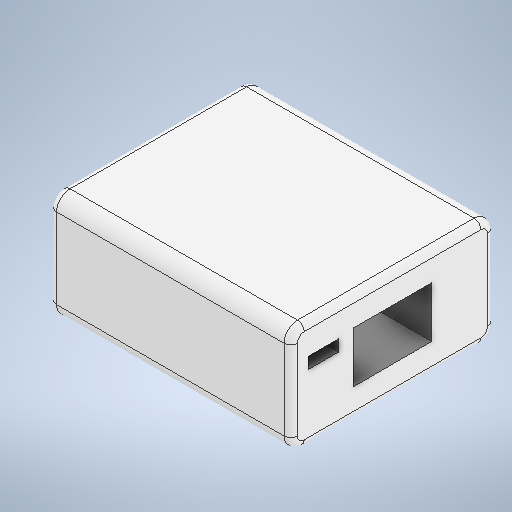
# Autodesk Inventor part: PoEbox
Saved by Autodesk Inventor 2025 (Build 290162000, 162)
## iProperties
Created: 2025-05-12
Part Number: PoEbox
Material: Generic
Document SubType Name: Modeling
Designer: ethan
Density: 1 g/cm^3
Appearance: Default(1)
Author: ethan
Autodesk Inventor part; units mm, degrees
ref_plane "YZ Plane" through (0, 0, 0) normal (1, 0, 0) x (0, 1, 0)
ref_plane "XZ Plane" through (0, 0, 0) normal (0, 1, 0) x (-1, 0, 0)
ref_plane "XY Plane" through (0, 0, 0) normal (0, 0, 1) x (1, 0, 0)
sketch "Sketch1" plane through (0, 0, 0) normal (0, 1, 0) x (-1, 0, 0)
  line L0 (0, 0) -> (57.15, 0)
  line L1 (57.15, 0) -> (57.15, -48.26)
  line L2 (57.15, -48.26) -> (0, -48.26)
  line L3 (0, -48.26) -> (0, 0)
  dimension "d0" = 57.15
  dimension "d1" = 48.26
  constraints: 8 end point, 2 parallel, 1 horizontal, 1 perpendicular
  measures "d0" distance of L1.end L2.end
  measures "d1" distance of L0.end L1.end
extrude "Extrusion1" add sketch "Sketch1" along normal blind 25.4
sketch "Sketch2" plane through (0, 0, 0) normal (1, 0, 0) x (0, 0, -1)
  line L0 (0, 0) -> (48.26, 0) construction
  line L1 (48.26, 0) -> (48.26, 25.4) construction
  line L2 (0, 25.4) -> (48.26, 25.4) construction
  line L3 (0, 0) -> (0, 25.4) construction
  line L4 (14.8042, 6.663) -> (33.4558, 6.663)
  line L5 (33.4558, 6.663) -> (33.4558, 18.737)
  line L6 (33.4558, 18.737) -> (14.8042, 18.737)
  line L7 (14.8042, 18.737) -> (14.8042, 6.663)
  line L8 (14.8042, 6.663) -> (33.4558, 18.737) construction
  line L9 (33.4558, 6.663) -> (14.8042, 18.737) construction
  line L10 (4.1311, 15.5562) -> (11.3642, 15.5562)
  line L11 (11.3642, 15.5562) -> (11.3642, 18.2577)
  line L12 (11.3642, 18.2577) -> (4.1311, 18.2577)
  line L13 (4.1311, 18.2577) -> (4.1311, 15.5562)
  line L14 (4.1311, 15.5562) -> (11.3642, 18.2577) construction
  line L15 (11.3642, 15.5562) -> (4.1311, 18.2577) construction
  point P0 (24.13, 12.7)
  point P1 (7.7477, 16.9069)
  constraints: 24 end point, 4 midpoint, 4 parallel, 2 horizontal, 2 perpendicular
extrude "Extrusion2" cut sketch "Sketch2" against normal blind 12.7
sketch "Sketch3" plane through (-57.15, 0, -48.26) normal (-1, 0, 0) x (0, 0, 1)
  line L0 (0, 0) -> (48.26, 0) projected
  line L1 (48.26, 0) -> (48.26, 25.4) projected
  line L2 (0, 25.4) -> (48.26, 25.4) projected
  line L3 (0, 0) -> (0, 25.4) projected
  circle A0 centre (24.13, 12.7) radius 2.54
  dimension "d6" = 5.08
  constraints: 1 centre point
  measures "d6" diameter of A0
extrude "Extrusion3" add sketch "Sketch3" along normal blind 7.62 contours A0
chamfer "Chamfer1" distance 0.254 distance2 7.62 1 edges at (-64.77, 12.7, -26.67) measured on face at (-64.77, 13.2614, -23.2922)
fillet "Fillet1" radius 3.175 4 edges at (-28.575, 25.4, -48.26) (-28.575, 0, -48.26) (-28.575, 0, 0) (-28.575, 25.4, 0)
fillet "Fillet2" radius 1.5875 18 edges at (0, 24.4701, -47.3301) (0, 12.7, -48.26) (0, 0.9299, -47.3301) (0, 0, -24.13) (0, 0.9299, -0.9299) (0, 12.7, 0) (0, 24.4701, -0.9299) (0, 25.4, -24.13) (-57.15, 24.4701, -0.9299) (-57.15, 12.7, 0) (-57.15, 0.9299, -0.9299) (-57.15, 0, -24.13) (-57.15, 0.9299, -47.3301) (-57.15, 12.7, -48.26) (-57.15, 24.4701, -47.3301) (-57.15, 25.4, -24.13) (-57.15, 12.7, -26.67) (-57.1505, 12.7, -26.67)
body "Solid1"
